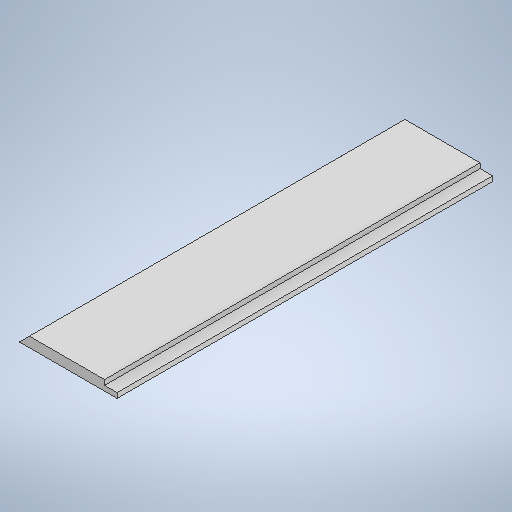
# Autodesk Inventor part: frontWallipt
Saved by Autodesk Inventor 2026.1 (Build 301233000, 233)
## iProperties
Created: 2026-08-16
Part Number: frontWallipt
Material: Generic
Document SubType Name: Modeling
Designer: rowan
Density: 1 g/cm^3
Appearance: Default
Author: rowan
Autodesk Inventor part; units mm, degrees
ref_plane "YZ Plane" through (0, 0, 0) normal (1, 0, 0) x (0, 1, 0)
ref_plane "XZ Plane" through (0, 0, 0) normal (0, 1, 0) x (-1, 0, 0)
ref_plane "XY Plane" through (0, 0, 0) normal (0, 0, 1) x (1, 0, 0)
sketch "Sketch1" plane through (0, 0, 0) normal (0, 1, 0) x (-1, 0, 0)
  line L0 (0, 0) -> (34.038, 0)
  line L1 (34.038, 0) -> (34.038, -150)
  line L2 (34.038, -150) -> (0, -150)
  line L3 (0, -150) -> (0, 0)
  line L4 (0, 0) -> (-5, 0)
  line L5 (-5, 0) -> (-5, -150)
  line L6 (-5, -150) -> (0, -150)
  dimension "d0" = 34.038
  dimension "d1" = 150
  dimension "d2" = 5
  constraints: 14 end point, 3 perpendicular, 2 horizontal, 2 parallel
  measures "d0" distance of L1.end L2.end
  measures "d1" distance of L0.end L1.end
  measures "d2" distance of L0.start L4.end
extrude "Extrusion1" add sketch "Sketch1" along normal blind 4 contours L0 L1 L2 L3
extrude "Extrusion2" add sketch "Sketch1" along normal blind 2 contours L3 L6 L5 L4
chamfer "Chamfer1" distance 4 angle 45 1 edges at (-34.038, 4, -75)
body "Solid1"
